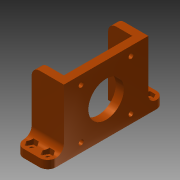
# Autodesk Inventor part: z motor mount
Saved by Autodesk Inventor 2014 (Build 180170000, 170)
## iProperties
Created: 2013-08-05
Part Number: z motor mount
Material: Generic
Document SubType Name: Modeling
Designer: employee
Density: 1 g/cm^3
Mass: 16.9502 g
Surface Area: 89.4267 cm^2
Volume: 16.9502 cm^3
Appearance: Smooth - Light Orange
Author: employee
Autodesk Inventor part; units mm, degrees
ref_plane "YZ Plane" through (0, 0, 0) normal (1, 0, 0) x (0, 1, 0)
ref_plane "XZ Plane" through (0, 0, 0) normal (0, 1, 0) x (-1, 0, 0)
ref_plane "XY Plane" through (0, 0, 0) normal (0, 0, 1) x (1, 0, 0)
sketch "Sketch1" plane through (0, 0, 0) normal (0, 0, 1) x (1, 0, 0)
  line L0 (0, -21.25) -> (0, 21.25)
  line L1 (0, 21.25) -> (-15, 21.25)
  line L2 (-15, 21.25) -> (-15, 26.25)
  line L3 (-15, 26.25) -> (5, 26.25)
  line L4 (5, 26.25) -> (5, -26.25)
  line L5 (5, -26.25) -> (-15, -26.25)
  line L6 (-15, -26.25) -> (-15, -21.25)
  line L7 (-15, -21.25) -> (0, -21.25)
  point P0 (0, 0)
  point P1 (0, 0)
  point P2 (5, 0)
  dimension "d0" = 42.5
  dimension "d2" = 5
  dimension "d3" = 5
  dimension "d4" = 20
  constraints: 16 end point, 5 parallel, 3 perpendicular, 2 midpoint, 1 coincident, 1 horizontal alignment, 1 vertical
  measures "d0" distance of L0.start L0.end
  measures "d2" distance between parallel lines of L4 L0
  measures "d3" distance of L1.end L2.end
  measures "d4" distance of L2.end L3.end
extrude "Extrusion1" add sketch "Sketch1" along normal blind 42
sketch "Sketch2" plane through (5, -26.25, 0) normal (1, 0, 0) x (0, 0, -1)
  line L0 (0, 52.5) -> (0, 0) projected
  line L1 (0, 52.5) -> (-42, 52.5) projected
  circle A0 centre (-21, 26.25) radius 11.05
  point P0 (0, 26.25)
  point P1 (0, 26.25)
  point P2 (-21, 52.5)
  dimension "d7" = 22.1
  constraints: 2 midpoint, 1 centre point, 1 horizontal alignment, 1 vertical alignment
  measures "d7" diameter of A0
extrude "Extrusion2" cut sketch "Sketch2" against normal through all
sketch "Sketch3" plane through (5, -26.25, 0) normal (1, 0, 0) x (0, 0, -1)
  circle A0 centre (-21, 26.25) radius 11.05 projected
  line L0 (-36.5, 41.75) -> (-5.5, 41.75)
  line L1 (-5.5, 41.75) -> (-5.5, 10.75)
  line L2 (-5.5, 10.75) -> (-36.5, 10.75)
  line L3 (-36.5, 10.75) -> (-36.5, 41.75)
  circle A1 centre (-36.5, 41.75) radius 1.55
  circle A2 centre (-5.5, 41.75) radius 1.55
  circle A3 centre (-5.5, 10.75) radius 1.55
  circle A4 centre (-36.5, 10.75) radius 1.55
  point P0 (0, 26.25)
  dimension "d11" = 31
  dimension "d12" = 3.1
  constraints: 8 end point, 5 coincident, 4 centre point, 3 equal radius, 1 horizontal, 9 other
  measures "d11" distance of L0.start L0.end
  measures "d12" diameter of A3
extrude "Extrusion3" cut sketch "Sketch3" against normal through all contours L3 A1 L0 | L0 A1 L3 | A2 L1 L0 | L0 L1 A2 | A4 L2 L3 | L3 L2 A4 | A3 L2 L1 | L1 L2 A3
sketch "Sketch4" plane through (-15, 26.25, 0) normal (0, 1, 0) x (1, 0, 0)
  line L0 (20, 0) -> (20, -42) projected
  line L1 (0, 0) -> (20, 0)
  line L2 (20, 0) -> (20, -5)
  line L3 (20, -5) -> (0, -5)
  line L4 (0, -5) -> (0, 0)
  point P0 (15, 0)
  dimension "d15" = 5
  constraints: 8 end point, 2 parallel, 1 horizontal, 1 perpendicular, 1 point on line
  measures "d15" distance between parallel lines of L1 L3
extrude "Extrusion4" add sketch "Sketch4" along normal blind 10
sketch "Sketch5" plane through (-15, -26.25, 0) normal (0, -1, 0) x (1, 0, 0)
  line L0 (20, 0) -> (0, 0) projected
  line L1 (20, 0) -> (20, 42) projected
  line L2 (0, 0) -> (20, 0)
  line L3 (20, 0) -> (20, 5)
  line L4 (20, 5) -> (0, 5)
  line L5 (0, 5) -> (0, 0)
  point P0 (15, 0)
  dimension "d19" = 5
  constraints: 8 end point, 2 parallel, 1 horizontal, 1 perpendicular, 1 point on line
  measures "d19" distance of L2.end L3.end
extrude "Extrusion5" add sketch "Sketch5" along normal blind 10
sketch "Sketch6" plane through (-15, 26.25, 5) normal (0, 0, 1) x (1, 0, 0)
  line L0 (20, 0) -> (0, 0) projected
  line L1 (20, 0) -> (20, 10) projected
  line L2 (0, 10) -> (20, 10) projected
  line L3 (0, -52.5) -> (20, -52.5) projected
  line L4 (0, -52.5) -> (0, -62.5) projected
  line L5 (20, -62.5) -> (0, -62.5) projected
  line L6 (20, -52.5) -> (20, -62.5) projected
  line L7 (5, 5) -> (15, 5)
  line L8 (5, -57.5) -> (15, -57.5)
  line L9 (0, -52.5) -> (20, -52.5) projected
  circle A0 centre (5, -57.5) radius 1.55
  circle A1 centre (15, -57.5) radius 1.55
  circle A2 centre (5, 5) radius 1.55
  circle A3 centre (15, 5) radius 1.55
  point P0 (15, -26.25)
  point P1 (20, 5)
  point P2 (20, -57.5)
  point P3 (10, 5)
  point P4 (10, 10)
  point P5 (10, -57.5)
  point P6 (10, -52.5)
  dimension "d26" = 5
  dimension "d27" = 3.1
  constraints: 6 midpoint, 4 centre point, 4 coincident, 4 end point, 3 equal radius, 3 parallel, 2 horizontal alignment, 2 vertical alignment, 1 perpendicular
  measures "d26" distance from line of L6 L8.end
  measures "d27" diameter of A0
extrude "Extrusion6" cut sketch "Sketch6" against normal through all contours A0 | A1 | A2 | A3
sketch "Sketch7" plane through (-15, 26.25, 5) normal (0, 0, 1) x (1, 0, 0)
  circle A0 centre (5, 5) radius 1.55 projected
  circle A1 centre (15, 5) radius 1.55 projected
  line L0 (8.2332, 5) -> (6.6166, 2.2)
  line L1 (6.6166, 2.2) -> (3.3834, 2.2)
  line L2 (3.3834, 2.2) -> (1.7668, 5)
  line L3 (1.7668, 5) -> (3.3834, 7.8)
  line L4 (3.3834, 7.8) -> (6.6166, 7.8)
  line L5 (6.6166, 7.8) -> (8.2332, 5)
  line L6 (18.2332, 5) -> (16.6166, 2.2)
  line L7 (16.6166, 2.2) -> (13.3834, 2.2)
  line L8 (13.3834, 2.2) -> (11.7668, 5)
  line L9 (11.7668, 5) -> (13.3834, 7.8)
  line L10 (13.3834, 7.8) -> (16.6166, 7.8)
  line L11 (16.6166, 7.8) -> (18.2332, 5)
  circle A2 centre (15, -57.5) radius 1.55 projected
  circle A3 centre (5, -57.5) radius 1.55 projected
  circle A4 centre (15, -57.5) radius 1.55 projected
  line L12 (0, -52.5) -> (20, -52.5) projected
  line L13 (0, -52.5) -> (0, -62.5) projected
  line L14 (20, -62.5) -> (0, -62.5) projected
  line L15 (20, -52.5) -> (20, -62.5) projected
  line L16 (8.2332, -57.5) -> (6.6166, -60.3)
  line L17 (6.6166, -60.3) -> (3.3834, -60.3)
  line L18 (3.3834, -60.3) -> (1.7668, -57.5)
  line L19 (1.7668, -57.5) -> (3.3834, -54.7)
  line L20 (3.3834, -54.7) -> (6.6166, -54.7)
  line L21 (6.6166, -54.7) -> (8.2332, -57.5)
  line L22 (11.7668, -57.5) -> (13.3834, -54.7)
  line L23 (13.3834, -54.7) -> (16.6166, -54.7)
  line L24 (16.6166, -54.7) -> (18.2332, -57.5)
  line L25 (18.2332, -57.5) -> (16.6166, -60.3)
  line L26 (16.6166, -60.3) -> (13.3834, -60.3)
  line L27 (13.3834, -60.3) -> (11.7668, -57.5)
  point P0 (15, -26.25)
  dimension "d31" = 5.6
  constraints: 48 end point, 4 coincident, 4 horizontal, 3 equal length, 52 other
  measures "d31" distance between parallel lines of L20 L17
extrude "Extrusion7" cut sketch "Sketch7" against normal blind 2.5 contours L0 L1 L2 L3 L4 L5 | L6 L7 L8 L9 L10 L11 | L16 L17 L18 L19 L20 L21 | L22 L23 L24 L25 L26 L27
fillet "Fillet1" radius 5 8 edges at (-5, -26.25, 5) (5, -36.25, 2.5) (-15, -36.25, 2.5) (-15, -23.75, 42) (-15, 23.75, 42) (-5, 26.25, 5) (5, 36.25, 2.5) (-15, 36.25, 2.5)
body "Solid1"
